Autodesk Fusion 360 part; units mm, degrees
(part 3 of 3)
  measures "d364" distance of L758.end L759.start
  measures "d365" distance of L758.end L758.start
  measures "d366" distance of L677.start L687.start
  measures "d367" distance of L701.end L687.start
  measures "d368" distance of L678.end L678.start
  measures "d369" distance of L678.start L685.end
  measures "d370" distance of L810.start L839.start
  measures "d371" distance of L817.end L839.start
  measures "d372" distance of L834.end L851.end
  measures "d373" distance of L834.end L834.start
  measures "d374" distance of L885.end L808.end
  measures "d375" distance of L808.start L808.end
  measures "d376" distance of L735.end L735.start
  measures "d377" distance of L725.end L735.start
  measures "d378" distance of L730.end L730.start
  measures "d379" distance of L730.start L727.end
  measures "d380" distance of L676.end L676.start
  measures "d381" distance of L683.end L676.start
  measures "d382" distance of L796.start L864.end
  measures "d383" distance of L849.end L864.end
  measures "d384" distance of L842.end L845.start
  measures "d385" distance of L784.end L842.end
  measures "d386" distance of L814.start L835.start
  measures "d387" distance of L772.end L835.start
  measures "d388" distance of L791.end L791.start
  measures "d389" distance of L832.start L791.start
  measures "d390" distance of L691.end L757.start
  measures "d391" distance of L691.end L691.start
  measures "d392" distance of L702.start L702.end
  measures "d393" distance of L702.start L756.start
  measures "d394" distance of L674.start L675.start
  measures "d395" distance of L693.end L675.start
  measures "d396" distance of L681.start L681.end
  measures "d397" distance of L681.start L690.end
  measures "d398" distance of L875.start L872.start
  measures "d399" distance of L875.start L863.end
  measures "d400" distance of L815.end L819.end
  measures "d401" distance of L815.end L815.start
  measures "d402" distance of L891.end L717.start
  measures "d403" distance of L672.end L891.end
  measures "d404" distance of L713.end L728.end
  measures "d405" distance of L713.end L713.start
  measures "d406" distance of L744.end L744.start
  measures "d407" distance of L743.end L744.start
  measures "d408" distance of L684.end L684.start
  measures "d409" distance of L750.start L684.start
  measures "d410" distance of L852.start L852.end
  measures "d411" distance of L852.start L797.end
  measures "d412" distance of L790.start L790.end
  measures "d413" distance of L790.start L803.end
  measures "d414" distance of L813.end L811.end
  measures "d415" distance of L811.end L811.start
  measures "d416" distance of L812.start L822.end
  measures "d417" distance of L822.end L822.start
  measures "d418" distance of L679.end L782.end
  measures "d419" distance of L679.start L679.end
  measures "d420" distance of L706.end L704.start
  measures "d421" distance of L706.end L706.start
  measures "d422" distance of L733.start L787.end
  measures "d423" distance of L787.end L787.start
  measures "d424" distance of L698.end L698.start
  measures "d425" distance of L720.end L698.start
  measures "d426" distance of L768.end L788.end
  measures "d427" distance of L768.end L768.start
  measures "d428" distance of L779.start L779.end
  measures "d429" distance of L779.start L848.start
  measures "d430" distance of L716.end L714.end
  measures "d431" distance of P17 L714.end
  measures "d432" distance of L724.end L715.end
  measures "d433" distance of P25 L715.end
  measures "d434" distance of L740.start L740.end
  measures "d435" distance of L740.start P15
  measures "d436" distance of L686.end L686.start
  measures "d437" distance of L686.start P12
  measures "d438" distance of L794.start L840.start
  measures "d439" distance of P16 L840.start
  measures "d440" distance of L764.start L764.end
  measures "d441" distance of P19 L764.start
  measures "d442" distance of L826.end L825.start
  measures "d443" distance of L826.end P22
  measures "d444" distance of L841.end L830.start
  measures "d445" distance of L841.end P21
  measures "d446" distance of L719.end L711.start
  measures "d447" distance of L719.end P13
  measures "d448" distance of L705.end L705.start
  measures "d449" distance of P20 L705.start
  measures "d450" distance of L694.start L773.start
  measures "d451" distance of P11 L773.start
  measures "d452" distance of L680.end L680.start
  measures "d453" distance of L680.start P18
  measures "d454" distance of L767.start L765.end
  measures "d455" distance of P6 L765.end
  measures "d456" distance of L785.start L786.start
  measures "d457" distance of P7 L786.start
  measures "d458" distance of L933.start L915.end
  measures "d459" distance of L915.start L915.end
  measures "d460" distance of L896.start L896.end
  measures "d461" distance of L919.end L896.start
  measures "d462" distance of L927.end L905.start
  measures "d463" distance of L927.end L918.end
  measures "d464" distance of L908.start L902.end
  measures "d465" distance of L902.end L902.start
  measures "d466" distance of L907.start L900.start
  measures "d467" distance of L907.start L917.start
  measures "d468" distance of L899.end L903.start
  measures "d469" distance of L899.start L899.end
  measures "d470" distance of L913.start L911.start
  measures "d471" distance of L913.start L897.end
  measures "d472" distance of L898.start L898.end
  measures "d473" distance of L898.start L906.end
  measures "d474" distance of L932.start L932.end
  measures "d475" distance of L932.start L934.end
  measures "d476" distance of L936.start L936.end
  measures "d477" distance of L931.end L936.start
  measures "d478" distance of L946.end L946.start
  measures "d479" distance of L929.end L946.start
  measures "d480" distance of L922.start L922.end
  measures "d481" distance of L922.start L924.end
  measures "d482" distance of L920.start L930.end
  measures "d483" distance of L930.start L930.end
  measures "d484" distance of L916.end L944.end
  measures "d485" distance of L916.end L916.start
  measures "d486" distance of L989.start L971.end
  measures "d487" distance of L971.start L971.end
  measures "d488" distance of L952.start L952.end
  measures "d489" distance of L975.end L952.start
  measures "d490" distance of L983.end L961.start
  measures "d491" distance of L983.end L974.end
  measures "d492" distance of L964.start L958.end
  measures "d493" distance of L958.end L958.start
  measures "d494" distance of L963.start L956.start
  measures "d495" distance of L963.start L973.start
  measures "d496" distance of L955.end L959.start
  measures "d497" distance of L955.start L955.end
  measures "d498" distance of L969.start L967.start
  measures "d499" distance of L969.start L953.end
  measures "d500" distance of L954.start L954.end
  measures "d501" distance of L954.start L962.end
  measures "d502" distance of L988.start L988.end
  measures "d503" distance of L988.start L990.end
  measures "d504" distance of L992.start L992.end
  measures "d505" distance of L987.end L992.start
  measures "d506" distance of L1002.end L1002.start
  measures "d507" distance of L985.end L1002.start
  measures "d508" distance of L978.start L978.end
  measures "d509" distance of L978.start L980.end
  measures "d510" distance of L976.start L986.end
  measures "d511" distance of L986.start L986.end
  measures "d512" distance of L972.end L1000.end
  measures "d513" distance of L972.end L972.start
  measures "d514" distance of L1008.start L1008.end
extrude "Extrude3" add sketch "Sketch4" against normal blind 2
extrude "Extrude4" cut 1 faces at (1.1667, 81, 38.3333) along direction (0, -1, 0) blind 1
ref_plane "WorkPlane3" through (1.5, 81, 1.5) normal (0, 1, 0) x (0, 0, 1)
sketch "Sketch6" plane through (1.5, 81, 1.5) normal (0, 1, 0) x (1, 0, 0)
  circle A0 centre (-1.5864, 1.3452) radius 34.9465 construction
  circle A1 centre (-1.5864, 1.3452) radius 34.4399
  circle A2 centre (-1.5864, 1.3452) radius 63.7618
  constraint concentric A0 A1
  constraint concentric A1 A2
extrude "Extrude5" cut sketch "Sketch6" against normal blind 44
